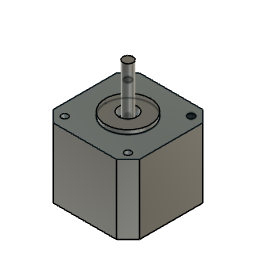
SM-42BYG v3 (Autodesk Fusion 360 design; units mm, degrees)
Autodesk Fusion 360 part; units mm, degrees
sketch "Sketch1" plane through (0, 0, 0) normal (0, 0, 1) x (1, 0, 0)
  line L0 (5.65, 0) -> (36.65, 0)
  line L1 (42.3, 5.65) -> (42.3, 36.65)
  line L2 (36.65, 42.3) -> (5.65, 42.3)
  line L3 (0, 36.65) -> (0, 5.65)
  line L4 (42.3, 36.65) -> (36.65, 42.3)
  line L5 (5.65, 42.3) -> (0, 36.65)
  line L6 (36.65, 0) -> (42.3, 5.65)
  line L7 (5.65, 0) -> (0, 5.65)
  dimension "d3" = 5.65
  dimension "d4" = 5.65
  dimension "d9" = 5.65
  constraint horizontal L0
  constraint vertical L1
  constraint horizontal L2
  constraint vertical L3
  constraint parallel L4 L7
  measures "d3" distance of L0 L1.start
  measures "d4" distance of L1 L0.end
  measures "d9" distance of origin L3.end
extrude "Extrude1" add sketch "Sketch1" along normal blind 34
sketch "Sketch2" plane through (0, 0, 34) normal (0, 0, 1) x (-1, 0, 0)
  line L0 (-36.65, 0) -> (-42.3, -5.65)
  line L1 (-42.3, -5.65) -> (-42.3, -36.65)
  line L2 (-42.3, -36.65) -> (-36.65, -42.3)
  line L3 (-36.65, -42.3) -> (-5.65, -42.3)
  line L4 (-5.65, -42.3) -> (0, -36.65)
  line L5 (0, -36.65) -> (0, -5.65)
  line L6 (0, -5.65) -> (-5.65, 0)
  line L7 (-5.65, 0) -> (-36.65, 0)
  circle A0 centre (-21.15, -21.15) radius 11
  circle A1 centre (-5.65, -36.65) radius 1.6
  circle A2 centre (-36.65, -36.65) radius 1.6
  dimension "d12" = 22
  dimension "d13" = 3.2
  dimension "d14" = 3.2
  dimension "d15" = 5.65
  dimension "d16" = 5.65
  dimension "d17" = 5.65
  dimension "d18" = 5.65
  dimension "d19" = 21.15
  dimension "d20" = 21.15
  measures "d12" diameter of A0
  measures "d13" diameter of A2
  measures "d14" diameter of A1
  measures "d15" distance of L5 A1.centre
  measures "d16" distance of L3 A1.centre
  measures "d17" distance of L3 A2.centre
  measures "d18" distance of L1 A2.centre
  measures "d19" distance of L5 A0.centre
  measures "d20" distance of L7 A0.centre
extrude "Extrude3" cut sketch "Sketch2" against normal blind 4.5 contours A1 | A2
extrude "Extrude2" add sketch "Sketch2" along normal blind 2 contours A0
pattern_linear "R-Pattern1" count 2 spacing 31 along (0, -1, 0) of "Extrude3"
sketch "Sketch3" plane through (0, 0, 36) normal (0, 0, 1) x (-1, 0, 0)
  circle A0 centre (-21.15, -21.15) radius 11
  circle A1 centre (-21.15, -21.15) radius 2.5
  dimension "d29" = 5
  constraint concentric A0 A1
  measures "d29" diameter of A1
extrude "Extrude4" add sketch "Sketch3" along normal blind 22 contours A1
sketch "Sketch4" plane through (0, 0, 36) normal (0, 0, 1) x (-1, 0, 0)
  circle A0 centre (-21.15, -21.15) radius 2.5
  circle A1 centre (-21.15, -21.15) radius 11
  circle A2 centre (-21.15, -21.15) radius 4.5
  dimension "d32" = 9
  constraint concentric A0 A2
  measures "d32" diameter of A2
extrude "Extrude5" cut sketch "Sketch4" against normal blind 4.5 contours A2
equation "d3 = ( 11.3 / 2 ) * 1 mm"
